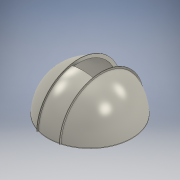
# Autodesk Inventor part: DomeHemisphere
Saved by Autodesk Inventor 2022 (Build 260153000, 153)
## iProperties
Created: 2021-05-07
Part Number: DomeHemisphere
Material: Generic
Document SubType Name: Modeling
Designer: Mick Veldhuis
Density: 1 g/cm^3
Appearance: Default
Author: Mick Veldhuis
Autodesk Inventor part; units mm, degrees
ref_plane "YZ Plane" through (0, 0, 0) normal (1, 0, 0) x (0, 1, 0)
ref_plane "XZ Plane" through (0, 0, 0) normal (0, 1, 0) x (-1, 0, 0)
ref_plane "XY Plane" through (0, 0, 0) normal (0, 0, 1) x (1, 0, 0)
sketch "Sketch1" plane through (0, 0, 0) normal (0, 1, 0) x (-1, 0, 0)
  circle A0 centre (0, 0) radius 3250
  circle A1 centre (0, 0) radius 3350
  dimension "d0" = 6500
  dimension "d1" = 6700
  constraints: 2 centre point, 2 coincident
  measures "d0" diameter of A0
  measures "d1" diameter of A1
extrude "Extrusion1" add sketch "Sketch1" along normal blind 50
sketch "Sketch2" plane through (0, 50, 0) normal (0, 1, 0) x (1, 0, 0)
  line L0 (0, -3350) -> (-920, -3350)
  line L1 (0, -3350) -> (920, -3350)
  line L2 (920, -3350) -> (920, -3221.1954)
  line L3 (-920, -3221.1954) -> (-920, -3350)
  line L4 (920, -3221.1954) -> (-920, -3221.1954)
  line L5 (0, 3350) -> (-920, 3350)
  line L6 (0, 3350) -> (920, 3350)
  line L7 (920, 3350) -> (920, 3221.1954)
  line L8 (-920, 3221.1954) -> (-920, 3350)
  line L9 (920, 3221.1954) -> (-920, 3221.1954)
  line L10 (920, 3221.1954) -> (920, -3221.1954)
  line L11 (-920, -3221.1954) -> (-920, 3221.1954)
  line L12 (3350, 0) -> (-3350, 0)
  line L13 (0, 3350) -> (0, -3350)
  line L14 (-920, 3117.0659) -> (920, 3117.0659)
  line L15 (-900, 3100) -> (-900, 3242)
  line L16 (-920, 3242) -> (-920, 3100)
  line L17 (900, 3100) -> (900, 3242)
  line L18 (920, 3242) -> (920, 3100)
  line L19 (-920, 3242) -> (-920, 3246)
  line L20 (-920, 3246) -> (-900, 3246)
  line L21 (-900, 3246) -> (-900, 3242)
  line L22 (-920, 3100) -> (-920, 3098)
  line L23 (920, 3100) -> (920, 3096)
  line L24 (920, 3096) -> (900, 3096)
  line L25 (900, 3096) -> (900, 3100)
  line L26 (900, 3242) -> (900, 3246)
  line L27 (900, 3246) -> (920, 3246)
  line L28 (920, 3246) -> (920, 3242)
  line L29 (-920, 3100) -> (-920, 3096)
  line L30 (-920, 3096) -> (-900, 3096)
  line L31 (-900, 3096) -> (-900, 3100)
  line L32 (-920, 3246) -> (-900, 3246)
  line L33 (-900, 3246) -> (-900, 3096)
  line L34 (-900, 3096) -> (-920, 3096)
  line L35 (-920, 3096) -> (-920, 3246)
  line L36 (900, 3246) -> (920, 3246)
  line L37 (920, 3246) -> (920, 3096)
  line L38 (920, 3096) -> (900, 3096)
  line L39 (900, 3096) -> (900, 3246)
  line L40 (-920, 3090) -> (-890, 3090)
  line L41 (-890, 3090) -> (-890, 3350)
  line L42 (-890, 3350) -> (-920, 3350)
  line L43 (-920, 3350) -> (-920, 3090)
  line L44 (920, 3090) -> (890, 3090)
  line L45 (890, 3090) -> (890, 3350)
  line L46 (890, 3350) -> (920, 3350)
  line L47 (920, 3350) -> (920, 3090)
  point P0 (0, 0)
  point P1 (0, 0)
  point P2 (-920, 0)
  point P3 (920, 0)
  point P4 (0, 0)
  point P5 (920, 0)
  point P6 (-920, 0)
  constraints: 96 end point, 15 parallel, 14 point on line, 8 horizontal, 7 coincident, 6 perpendicular, 2 midpoint, 2 vertical
ref_plane "Work Plane1" through (0, 50, -3350) normal (-1, 0, 0) x (0, 0, 1)
sketch3d "DomeSketch"
ref_plane "Work Plane2" through (0, 50, 0) normal (0, 1, 0) x (1, 0, 0)
sketch "Sketch3" plane through (0, 50, 0) normal (0, 1, 0) x (1, 0, 0)
  circle A0 centre (0, 0) radius 3350 projected
  line L0 (0, 3350) -> (0, -3350)
  constraints: 2 end point, 2 point on circle, 1 coincident, 1 vertical
sketch3d "3D Sketch2"
sketch "Sketch4" plane through (0, 50, -3350) normal (-1, 0, 0) x (0, 0, 1)
  arc A0 (3350, 3350) -> (0, 0) centre (3350, 0) ccw
  arc A1 (3350, 3250) -> (100, 0) centre (3350, 0) ccw
  line L0 (3350, 3350) -> (3350, 3250)
  line L1 (0, 0) -> (100, 0)
  line L2 (6700, -50) -> (0, -50) projected
  line L3 (3350, 3250) -> (3350, 0)
  line L4 (3350, 0) -> (100, 0)
  point P0 (3350, -50)
  constraints: 8 end point, 4 point on circle, 2 centre point, 2 vertical, 1 coincident, 1 parallel, 1 perpendicular
revolve "Revolution1" add sketch "Sketch4" angle 360 about axis through (0, 3400, 0) along (0, -1, 0) contours L0 A1 L1 A0
sketch3d "3D Sketch3"
revolve "Revolution2" cut sketch "Sketch2" angle 100 about axis through (3350, 50, 0) along (1, 0, 0) contours L14 L41 L9 L13 | L13 L9 L45 L14 | L13 L6 L45 L9 | L9 L41 L5 L13 | L14 L15 L9 L41 | L45 L9 L17 L14 | L45 L6 L7 L27 L26 L17 L9 | L9 L15 L21 L20 L8 L5 L41 | L14 L11 L9 L15 | L17 L9 L10 L14 | L17 L26 L27 L7 L9 | L9 L8 L20 L21 L15
sketch "Sketch5" plane through (0, 50, 0) normal (0, 0.1736482, -0.9848078) x (-1, 0, 0)
  arc A0 (920, 3221.1954) -> (-920, 3221.1954) centre (0, 0) ccw projected
  arc A1 (920, 3117.0659) -> (-920, 3117.0659) centre (0, 0) ccw projected
  line L0 (-920, 3221.1954) -> (-920, 3117.0659)
  line L1 (920, -559.3547) -> (920, 3221.1954) projected
  line L2 (920, 3221.1954) -> (920, 3117.0659)
  point P0 (0, -49.2404)
  constraints: 4 end point, 1 collinear, 1 vertical
revolve "Revolution3" add sketch "Sketch2" angle 180 about axis through (3350, 50, 0) along (1, 0, 0) contours L11 L30 L31 L15 L14 L41 L40 | L44 L45 L14 L17 L25 L24 L10 | L14 L15 L9 L41 | L45 L9 L17 L14 | L11 L14 L15 L31 L30 | L24 L25 L17 L14 L10 | L45 L6 L7 L27 L26 L17 L9 | L9 L15 L21 L20 L8 L5 L41 | L14 L11 L9 L15 | L17 L9 L10 L14 | L17 L26 L27 L7 L9 | L9 L8 L20 L21 L15
body "Solid1"
